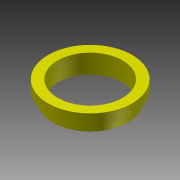
# Autodesk Inventor part: Regulator Ring 2 1764
Saved by Autodesk Inventor 2011 (Build 150239000, 239)
## iProperties
Created: 2010-02-17
Part Number: Regulator Ring 2 1764
Document SubType Name: Modeling
Designer: jgehrig
Density: 1 g/cm^3
Author: jgehrig
Autodesk Inventor part; units mm, degrees
ref_plane "YZ Plane" through (0, 0, 0) normal (1, 0, 0) x (0, 1, 0)
ref_plane "XZ Plane" through (0, 0, 0) normal (0, 1, 0) x (-1, 0, 0)
ref_plane "XY Plane" through (0, 0, 0) normal (0, 0, 1) x (1, 0, 0)
sketch "Sketch1" plane through (0, 0, 0) normal (0, 0, 1) x (1, 0, 0)
  line L0 (-27.1692, 18.0644) -> (-23.9942, 18.0644)
  line L1 (-23.9942, 18.0644) -> (-23.9942, 11.7144)
  line L2 (-23.9942, 11.7144) -> (-25.5817, 11.7144)
  line L3 (-25.5817, 11.7144) -> (-25.5817, 14.8894)
  line L4 (-25.5817, 14.8894) -> (-27.1692, 14.8894)
  line L5 (-27.1692, 14.8894) -> (-27.1692, 18.0644)
  line L6 (-13.1992, 23.4202) -> (-13.1992, 2.3302)
  point P0 (0, 0)
  dimension "d0" = 3.175
  dimension "d1" = 3.175
  dimension "d4" = 13.97
  dimension "d6" = 3.175
  constraints: 14 end point, 6 parallel, 1 horizontal, 1 perpendicular
  measures "d0" distance of L4.end L0.start
  measures "d1" distance of L2.end L3.end
  measures "d4" distance between parallel lines of L6 L5
  measures "d6" distance of L0.start L0.end
revolve "Revolution1" add sketch "Sketch1" angle 360 about axis through (-13.1992, 23.4202, 0) along (0, -1, 0)
body "Solid1"
